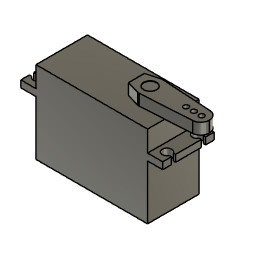
Servomotor - DS5160 v4 (Autodesk Fusion 360 design; units mm, degrees)
Autodesk Fusion 360 part; units mm, degrees
note: some values were not read from the file. Set by a fixed rule: which sketch regions a step uses.
sketch "Skizze1" plane through (0, 0, 0) normal (0, 0, 1) x (1, 0, 0)
  line L0 (-35, 20) -> (30, 20)
  line L1 (30, 20) -> (30, -10)
  line L2 (30, -10) -> (-35, -10)
  line L3 (-35, -10) -> (-35, 20)
  dimension "d1" = 65
  dimension "d2" = 30
  constraint horizontal L0
  constraint vertical L1
  constraint horizontal L2
  constraint vertical L3
  measures "d1" distance of L0.start L0.end
  measures "d2" distance of L0 L2
extrude "Extrusion1" add sketch "Skizze1" along normal blind 47.8 makes body 1
sketch "Skizze4" plane through (-35, 0, 0) normal (-1, 0, 0) x (0, -1, 0)
  line L0 (-20, 0) -> (10, 0)
  line L1 (10, 0) -> (10, 47.8)
  line L2 (10, 47.8) -> (-20, 47.8)
  line L3 (-20, 47.8) -> (-20, 0)
  line L4 (-20, 35.7) -> (10, 35.7)
  line L5 (10, 35.7) -> (10, 31.7)
  line L6 (10, 31.7) -> (-20, 31.7)
  line L7 (-20, 31.7) -> (-20, 35.7)
  line L8 (10, 0) -> (-20, 0)
  line L9 (10, 35.7) -> (-20, 35.7)
  line L10 (-20, 35.7) -> (-20, 31.7)
  line L11 (-20, 31.7) -> (10, 31.7)
  line L12 (10, 31.7) -> (10, 35.7)
  dimension "d7" = 4
  dimension "d8" = 31.7
  constraint horizontal L4
  constraint vertical L5
  constraint horizontal L6
  constraint vertical L7
  constraint coincident L1 L5.end
  constraint coincident L3 L4.start
  constraint horizontal L9
  constraint vertical L10
  constraint horizontal L11
  constraint vertical L12
  measures "d7" distance of L4 L6
  measures "d8" distance of L6 L8
sketch "Skizze5" plane through (30, 0, 0) normal (1, 0, 0) x (0, 1, 0)
  line L0 (-10, 0) -> (20, 0)
  line L1 (20, 0) -> (20, 47.8)
  line L2 (20, 47.8) -> (-10, 47.8)
  line L3 (-10, 47.8) -> (-10, 0)
  line L4 (-10, 35.7) -> (20, 35.7)
  line L5 (20, 35.7) -> (20, 31.7)
  line L6 (20, 31.7) -> (-10, 31.7)
  line L7 (-10, 31.7) -> (-10, 35.7)
  line L8 (20, 0) -> (-10, 0)
  dimension "d9" = 4
  dimension "d10" = 31.7
  constraint horizontal L4
  constraint vertical L5
  constraint horizontal L6
  constraint vertical L7
  constraint coincident L1 L5.end
  constraint coincident L3 L4.start
  measures "d9" distance of L4 L6
  measures "d10" distance of L6 L8
extrude "Extrusion2" add sketch "Skizze4" along normal blind 8.8 contours L1 L3 L4 L5 L6 L7 L9 L10 L11 L12 bodies 1
extrude "Extrusion3" add sketch "Skizze5" along normal blind 8.8 contours L1 L3 L4 L5 L6 L7 bodies 1
copy_body "Körper->Berechn1" bodies 1 removing the originals makes body 2 in component "Corpus"
sketch "Skizze6" plane through (0, 0, 47.8) normal (0, 0, 1) x (-1, 0, 0)
  line L0 (35, 10) -> (-30, 10)
  line L1 (-30, 10) -> (-30, -20)
  line L2 (-30, -20) -> (35, -20)
  line L3 (35, -20) -> (35, 10)
  line L4 (-8.5, 10) -> (-8.5, -20) construction
  line L5 (35, 10) -> (35, -20)
  line L6 (-16.5, 10) -> (-16.5, -20) construction
  line L7 (-30, -5) -> (-7, -5) construction
  line L8 (-30, 10) -> (35, 10) construction
  circle A0 centre (-16.5, -5) radius 2.5
  circle A1 centre (-16.5, -5) radius 8.75 construction
  dimension "d15" = 43.5
  dimension "d16" = 8
  dimension "d17" = 15
  dimension "d18" = 5
  dimension "d19" = 17.5
  constraint coincident L0 L4.start
  constraint coincident L2 L4.end
  constraint perpendicular L2 L4
  constraint coincident L0 L6.start
  constraint perpendicular L0 L6
  constraint coincident L1 L7.start
  constraint perpendicular L4 L7
  constraint midpoint L6 A0.centre
  constraint concentric A0 A1
  measures "d15" distance of L4 L5
  measures "d16" distance of L4 L6
  measures "d17" distance of L7 L8
  measures "d18" diameter of A0
  measures "d19" diameter of A1
extrude "Extrusion1'" add sketch "Skizze6" along normal blind 1 separate body contours A0 makes body 3 in component "Corpus"
sketch "Skizze7" plane through (0, 0, 47.8) normal (0, 0, 1) x (-1, 0, 0)
  line L0 (35, 10) -> (-30, 10)
  line L1 (-30, -20) -> (35, -20)
  line L2 (35, -20) -> (35, 10)
  line L3 (-51, 7) -> (-51, -5.0519) construction
  line L4 (-20, 1.9) -> (-13, 1.9) construction
  line L5 (-20, -11.9) -> (-13, -11.9) construction
  line L6 (-10, -0.35) -> (-7, -0.35) construction
  line L7 (-10, -9.65) -> (-7, -9.65) construction
  line L8 (-53, -0.25) -> (-49, -0.25) construction
  line L9 (-53, -9.75) -> (-49, -9.75) construction
  line L10 (-46.311, -10.0422) -> (-17.0084, -11.8683)
  line L11 (-46.311, 0.0422) -> (-17.0084, 1.8683)
  line L12 (-16.0096, 1.7621) -> (-8.5, -0.35)
  line L13 (-16.0096, -11.7621) -> (-8.5, -9.65)
  line L14 (-8.5, -0.35) -> (-8.5, -9.65)
  arc A0 (-51, -5.0519) -> (-46.311, -10.0422) centre (-46, -5.0519) ccw
  arc A1 (-46.311, 0.0422) -> (-51, -4.9481) centre (-46, -4.9481) ccw
  arc A2 (-17.0084, -11.8683) -> (-16.0096, -11.7621) centre (-16.8218, -8.8741) ccw
  arc A3 (-16.0096, 1.7621) -> (-17.0084, 1.8683) centre (-16.8218, -1.1259) ccw
  line L15 (-51, -4.9481) -> (-51, -5.0519)
  circle A4 centre (-16.5, -5) radius 2.5
  point P0 (-16.5, -5)
  dimension "d22" = 34.5
  dimension "d23" = 13.8
  dimension "d24" = 6.9
  dimension "d25" = 9.3
  dimension "d26" = 4.65
  dimension "d27" = 9.5
  dimension "d28" = 4.75
  dimension "d29" = 5
  dimension "d30" = 5
  dimension "d31" = 3
  dimension "d32" = 3
  dimension "d36" = 5
  constraint vertical L3
  constraint parallel L0 L4
  constraint horizontal L6
  constraint perpendicular L3 L8
  constraint horizontal L9
  constraint midpoint L6 L12.end
  constraint midpoint L7 L13.end
  constraint perpendicular L7 L14
  constraint tangent L10 A0
  constraint tangent L3 A0
  constraint tangent L11 A1
  constraint tangent L10 A2
  constraint tangent L13 A2
  constraint tangent L11 A3
  constraint tangent L12 A3
  constraint tangent A0 L15
  constraint coincident P0 A4.centre
  measures "d22" distance of L3 P0
  measures "d23" distance of L4 L5
  measures "d24" distance of P0 L5
  measures "d25" distance of L6 L7
  measures "d26" distance of P0 L7
  measures "d27" distance of L8 L9
  measures "d28" distance of P0 L9
  measures "d29" radius of A0
  measures "d30" radius of A1
  measures "d31" radius of A2
  measures "d32" radius of A3
  measures "d36" diameter of A4
extrude "Extrusion4" add sketch "Skizze7" along normal blind 6.5 from surface at 1 separate body contours L10 L11 L12 L13 L14 A0 A1 A2 A3 L15 | A4 makes body 4
copy_body "Körper->Berechn2" bodies 4 removing the originals makes body 5 in component "Konnektor"
sketch "Skizze8" plane through (0, 0, 55.3) normal (0, 0, 1) x (-1, 0, 0)
  arc A0 (-46.311, 0.0422) -> (-51, -4.9481) centre (-46, -4.9481) ccw
  line L0 (-51, -4.9481) -> (-51, -5.0519)
  arc A1 (-51, -5.0519) -> (-46.311, -10.0422) centre (-46, -5.0519) ccw
  line L1 (-46.311, -10.0422) -> (-17.0084, -11.8683)
  arc A2 (-17.0084, -11.8683) -> (-16.0096, -11.7621) centre (-16.8218, -8.8741) ccw
  line L2 (-16.0096, -11.7621) -> (-8.5, -9.65)
  line L3 (-8.5, -9.65) -> (-8.5, -0.35)
  line L4 (-8.5, -0.35) -> (-16.0096, 1.7621)
  arc A3 (-16.0096, 1.7621) -> (-17.0084, 1.8683) centre (-16.8218, -1.1259) ccw
  line L5 (-17.0084, 1.8683) -> (-46.311, 0.0422)
  circle A4 centre (-16.5, -5) radius 2.5
  dimension "d41" = 5
  measures "d41" diameter of A4
sketch "Skizze9" plane through (0, 0, 35.7) normal (0, 0, 1) x (-1, 0, 0)
  line L0 (-30, -20) -> (-30, 10)
  line L1 (-30, 10) -> (-38.8, 10)
  line L2 (-38.8, 10) -> (-38.8, -20)
  line L3 (-38.8, -20) -> (-30, -20)
  circle A0 centre (-35.05, -13.75) radius 2.75
  line L4 (-38.8, -5) -> (-30, -5) construction
  circle A1 centre (-35.05, 3.75) radius 2.75
  line L5 (-38.8, -12.5) -> (-37.8, -12.5)
  line L6 (-37.8, -15) -> (-38.8, -15)
  line L7 (-38.8, -15) -> (-38.8, -12.5)
  line L8 (-38.8, -13.75) -> (-37.5, -13.75) construction
  line L9 (-37.8, -12.5) -> (-37, -12.5)
  line L10 (-37, -12.5) -> (-37, -15)
  line L11 (-37, -15) -> (-37.8, -15)
  line L12 (-37.8, 5) -> (-38.8, 5)
  line L13 (-38.8, 5) -> (-38.8, 2.5)
  line L14 (-38.8, 2.5) -> (-37.8, 2.5)
  line L15 (-37, 2.5) -> (-37, 5)
  line L16 (-37, 5) -> (-37.8, 5)
  line L17 (-37.8, 2.5) -> (-37, 2.5)
  line L18 (2.5, 10) -> (2.5, -20) construction
  circle A2 centre (40.05, 3.75) radius 2.75
  line L19 (42.8, 5) -> (43.8, 5)
  line L20 (43.8, 5) -> (43.8, 2.5)
  line L21 (42.8, 2.5) -> (42, 2.5)
  line L22 (42, 2.5) -> (42, 5)
  line L23 (42, 5) -> (42.8, 5)
  line L24 (43.8, 2.5) -> (42.8, 2.5)
  circle A3 centre (40.05, -13.75) radius 2.75
  line L25 (42.8, -15) -> (43.8, -15)
  line L26 (43.8, -15) -> (43.8, -12.5)
  line L27 (43.8, -12.5) -> (42.8, -12.5)
  line L28 (42.8, -12.5) -> (42, -12.5)
  line L29 (42, -15) -> (42.8, -15)
  line L30 (42, -12.5) -> (42, -15)
  dimension "d46" = 5.5
  dimension "d50" = 6.25
  dimension "d51" = 2.5
  dimension "d54" = 6.25
  dimension "d56" = 1.25
  dimension "d57" = 41.3
  constraint midpoint L2 L4.start
  constraint perpendicular L2 L4
  constraint symmetric A0 L4 A1
  constraint horizontal L5
  constraint horizontal L6
  constraint vertical L7
  constraint coincident L2 L5.start
  constraint coincident L2 L8.start
  constraint horizontal L9
  constraint vertical L10
  constraint horizontal L11
  constraint symmetric L4 L5.start L13.end
  constraint symmetric L4 L5.end L14.end
  constraint symmetric L4 L6.start L12.start
  constraint symmetric L4 L6.end L12.end
  constraint symmetric L4 L9.end L15.start
  constraint symmetric L4 L10.end L15.end
  constraint vertical L18
  constraint symmetric A0 L18 A3
  constraint symmetric A1 L18 A2
  constraint symmetric L5.start L18 L26.end
  constraint symmetric L5.end L18 L27.end
  constraint symmetric L6.start L18 L25.start
  constraint symmetric L6.end L18 L25.end
  constraint symmetric L9.end L18 L28.end
  constraint symmetric L10.end L18 L29.start
  constraint symmetric L12.start L18 L19.start
  constraint symmetric L12.end L18 L19.end
  constraint symmetric L13.end L18 L20.end
  constraint symmetric L14.end L18 L21.start
  constraint symmetric L15.start L18 L21.end
  constraint symmetric L15.end L18 L22.end
  measures "d46" diameter of A0
  measures "d50" distance of L3 A0.centre
  measures "d51" distance of L5 L6
  measures "d54" distance of L3 L8
  measures "d56" distance of L5 L8
  measures "d57" distance of L2 L18
extrude "Extrusion2'" cut sketch "Skizze9" against normal blind 5 contours L2 A0 L5 L6 L7 L9 L11 | L2 A1 L12 L13 L14 L16 L17 | A0 L9 L10 L11 | A0 L9 L10 L11 | A1 L15 L16 L17 | A1 L15 L16 L17 | A2 L21 L22 L23 | A2 L19 L20 L21 L23 L24 | A2 L21 L22 L23 | A3 L28 L29 L30 | A3 L25 L26 L27 L28 L29 | A3 L28 L29 L30 bodies 2 in component "Corpus"
sketch "Skizze10" plane through (0, 0, 55.3) normal (0, 0, 1) x (-1, 0, 0)
  arc A0 (-46.311, 0.0422) -> (-51, -4.9481) centre (-46, -4.9481) ccw
  line L0 (-51, -4.9481) -> (-51, -5.0519)
  arc A1 (-51, -5.0519) -> (-46.311, -10.0422) centre (-46, -5.0519) ccw
  line L1 (-46.311, -10.0422) -> (-17.0084, -11.8683)
  arc A2 (-17.0084, -11.8683) -> (-16.0096, -11.7621) centre (-16.8218, -8.8741) ccw
  line L2 (-16.0096, -11.7621) -> (-8.5, -9.65)
  line L3 (-8.5, -9.65) -> (-8.5, -0.35)
  line L4 (-8.5, -0.35) -> (-16.0096, 1.7621)
  arc A3 (-16.0096, 1.7621) -> (-17.0084, 1.8683) centre (-16.8218, -1.1259) ccw
  line L5 (-17.0084, 1.8683) -> (-46.311, 0.0422)
  circle A4 centre (-46.5, -5) radius 1.5
  line L6 (-51, 0) -> (-51, -10.2733) construction
  circle A5 centre (-42, -5) radius 1.5
  circle A6 centre (-37.5, -5) radius 1.5
  circle A7 centre (-16.5, -5) radius 3.75
  dimension "d61" = 3
  dimension "d62" = 4.5
  dimension "d63" = 3
  dimension "d64" = 4.5
  dimension "d65" = 3
  dimension "d66" = 4.5
  dimension "d69" = 7.5
  constraint vertical L6
  measures "d61" diameter of A4
  measures "d62" distance of A4.centre L6
  measures "d63" diameter of A5
  measures "d64" distance of A4.centre A5.centre
  measures "d65" diameter of A6
  measures "d66" distance of A5.centre A6.centre
  measures "d69" diameter of A7
extrude "Extrusion1''" cut sketch "Skizze10" against normal blind 8 contours A4 | A5 | A6 bodies 5 in component "Konnektor"
extrude "Extrusion2''" cut sketch "Skizze10" against normal blind 0.25 contours A7 bodies 5 in component "Konnektor"
component "Corpus" placed x (1, 0, 0) y (0, 1, 0) z (0, 0, 1) at (0, 0, 0)
component "Konnektor" placed x (1, 0, 0) y (0, 1, 0) z (0, 0, 1) at (0, 0, 0)
named bodies: "Corpus", "Drehgelenk", "Konnektor"
